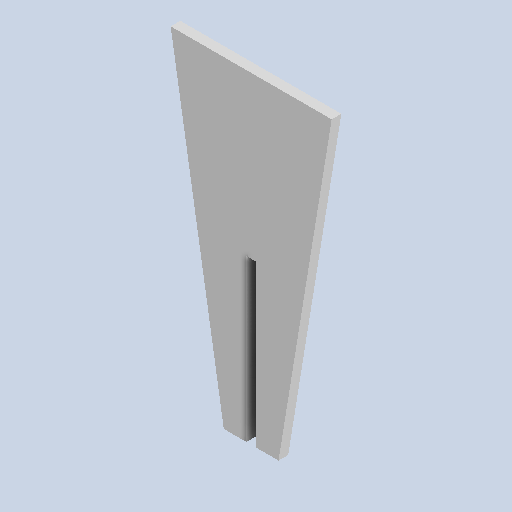
# Autodesk Inventor part: Base_Estructura
Saved by Autodesk Inventor 2022 (Build 260153000, 153)
## iProperties
Created: 2022-01-30
Part Number: Base_Estructura
Material: Generic
Document SubType Name: Modeling
Designer: katha
Density: 1 g/cm^3
Appearance: Default
Author: katha
Autodesk Inventor part; units mm, degrees
ref_plane "YZ Plane" through (0, 0, 0) normal (1, 0, 0) x (0, 1, 0)
ref_plane "XZ Plane" through (0, 0, 0) normal (0, 1, 0) x (-1, 0, 0)
ref_plane "XY Plane" through (0, 0, 0) normal (0, 0, 1) x (1, 0, 0)
sketch "Sketch1" plane through (0, 0, 0) normal (0, 0, 1) x (1, 0, 0)
  line L0 (1.5, 216.5) -> (-1.5, 216.5) projected
  line L1 (0, 216.5) -> (-25, 216.5)
  line L2 (-1.5, 116.5) -> (-8.5, 116.5)
  line L3 (-8.5, 116.5) -> (-25, 216.5)
  line L4 (-1.5, 116.5) -> (-1.5, 166.5)
  line L5 (-1.5, 166.5) -> (0, 166.5)
  line L6 (0, 166.5) -> (0, 216.5) construction
  line L7 (0, 216.5) -> (25, 216.5)
  line L8 (1.5, 116.5) -> (8.5, 116.5)
  line L9 (8.5, 116.5) -> (25, 216.5)
  line L10 (1.5, 116.5) -> (1.5, 166.5)
  line L11 (1.5, 166.5) -> (0, 166.5)
  point P0 (0, 0)
  dimension "d0" = 25
  dimension "d6" = 8.5
  dimension "d7" = 99.369
  dimension "d8" = 50
  dimension "d9" = 1.5
  dimension "d10" = 50
  constraints: 22 end point, 4 symmetric about line, 2 horizontal, 2 vertical, 1 midpoint
  measures "d0" distance of L1.start L1.end
  measures "d6" distance from line of L2.end L6
  measures "d7" angle of L3 L1
  measures "d8" distance from line of L1 L5.end
  measures "d9" distance of L4.end L5.end
  measures "d10" distance of L2.start L4.end
extrude "Extrusion1" add sketch "Sketch1" along normal blind 3
body "Solid1"
